Ikea Schienen Verbinder (Autodesk Fusion 360 design; units mm, degrees)
Autodesk Fusion 360 part; units mm, degrees
sketch "Sketch1" plane through (0, 0, 0) normal (0, 0, 1) x (1, 0, 0)
  line L0 (0, 0) -> (12.9, 0)
  line L1 (12.9, 0) -> (12.9, 50)
  line L2 (12.9, 50) -> (0, 50)
  line L3 (0, 50) -> (0, 0)
  dimension "d1" = 12.9
  dimension "d2" = 50
  constraint horizontal L0
  constraint vertical L1
  constraint horizontal L2
  constraint vertical L3
  constraint coincident L0.start L3.end
  measures "d1" distance of L0.start L0.end
  measures "d2" distance of L0.start L2.end
extrude "Extrude1" add sketch "Sketch1" along normal blind 6.5
chamfer "Chamfer1" distance 9 distance2 3 2 edges at (0, 0, 3.25) (12.9, 50, 3.25) measured on face at (0, 33.3333, 4.3333) measured on face at (12.9, 16.6667, 4.3333)
chamfer "Chamfer2" distance 3 distance2 9 2 edges at (12.9, 0, 3.25) (0, 50, 3.25) measured on face at (6.3, 0, 2.1667) measured on face at (6.6, 50, 2.1667)
chamfer "Chamfer3" distance 9 distance2 3 1 edges at (6.45, 50, 6.5) measured on face at (4.3, 19.6667, 6.5)
chamfer "Chamfer4" distance 9 distance2 3 1 edges at (6.45, 0, 6.5) measured on face at (4.3, 30.3333, 6.5)
equation "d5 = splinter"
equation "d8 = splinter"
equation "d9 = splinter"
equation "d11 = splinter"
equation "splinter = 9 mm"
